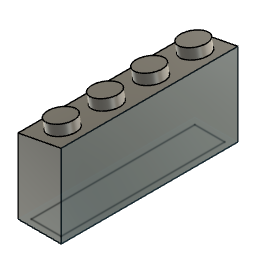
lego_1x4_pfeiler v3 (Autodesk Fusion 360 design; units mm, degrees)
Autodesk Fusion 360 part; units mm, degrees
sketch "Skizze1" plane through (0, 0, 0) normal (0, 0, 1) x (1, 0, 0)
  line L0 (-3.9, -16) -> (3.9, -16)
  line L1 (3.9, -16) -> (3.9, 16)
  line L2 (3.9, 16) -> (-3.9, 16)
  line L3 (-3.9, 16) -> (-3.9, -16)
  line L4 (-3.9, -16) -> (3.9, 16) construction
  line L5 (3.9, -16) -> (-3.9, 16) construction
  dimension "d1" = 7.8
  dimension "d2" = 32
  constraint horizontal L0
  constraint perpendicular L0 L1
  constraint parallel L0 L2
  constraint parallel L1 L3
  constraint coincident L4 origin
  constraint coincident L5 origin
  measures "d1" distance of L1.end L2.end
  measures "d2" distance of L0.end L1.end
extrude "Extrusion1" add sketch "Skizze1" along normal blind 15
sketch "Skizze2" plane through (3.9, 0, 0) normal (1, 0, 0) x (0, 1, 0)
  line L0 (-16, 0) -> (16, 0)
  line L1 (16, 0) -> (16, 15)
  line L2 (16, 15) -> (-16, 15)
  line L3 (-16, 15) -> (-16, 0)
sketch "Skizze3" plane through (0, -16, 0) normal (0, -1, 0) x (1, 0, 0)
  line L0 (-3.9, 0) -> (3.9, 0)
  line L1 (3.9, 0) -> (3.9, 15)
  line L2 (3.9, 15) -> (-3.9, 15)
  line L3 (-3.9, 15) -> (-3.9, 0)
  line L4 (3.9, 15) -> (-3.9, 13.511)
  dimension "d19" = 13.511
  constraint coincident L1.end L2.start
  constraint coincident L3 L4.end
  measures "d19" distance of L0.start L4.end
extrude "Extrusion2" cut sketch "Skizze3" against normal through all contours L2 L3 L4
sketch "Skizze4" plane through (-2.6257, 0, 13.7543) normal (-0.187511, 0, 0.982262) x (0, -1, 0)
  line L0 (-16, 6.6435) -> (-16, -1.2974)
  line L1 (-16, -1.2974) -> (16, -1.2974)
  line L2 (16, -1.2974) -> (16, 6.6435)
  line L3 (16, 6.6435) -> (-16, 6.6435)
  circle A0 centre (-12.1, 2.7435) radius 2.4
  circle A1 centre (-4.1, 2.7435) radius 2.4
  circle A2 centre (3.9, 2.7435) radius 2.4
  circle A3 centre (11.9, 2.7435) radius 2.4
  dimension "d6" = 4.8
  dimension "d7" = 3.9
  dimension "d8" = 3.9
  dimension "d11" = 8
  dimension "d12" = 0
  measures "d6" diameter of A0
  measures "d7" distance of L0 A0.centre
  measures "d8" distance of L3 A0.centre
extrude "Extrusion3" add sketch "Skizze4" along normal blind 1.8 contours A0 | A1 | A2 | A3
sketch "Skizze5" plane through (0, 0, 0) normal (0, 0, -1) x (1, 0, 0)
  line L0 (-3.9, 16) -> (-3.9, -16)
  line L1 (-3.9, -16) -> (3.9, -16)
  line L2 (3.9, -16) -> (3.9, 16)
  line L3 (3.9, 16) -> (-3.9, 16)
  line L4 (-2.7, 14.8) -> (-2.7, -14.8)
  line L5 (-2.7, -14.8) -> (2.7, -14.8)
  line L6 (2.7, -14.8) -> (2.7, 14.8)
  line L7 (2.7, 14.8) -> (-2.7, 14.8)
  dimension "d15" = -1.2
extrude "Extrusion4" cut sketch "Skizze5" against normal blind 11 contours L4 L5 L6 L7
